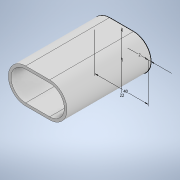
# Autodesk Inventor part: round
Saved by Autodesk Inventor 2022 (Build 260153000, 153)
## iProperties
Created: 2021-10-11
Part Number: round
Material: Generic
Document SubType Name: Modeling
Designer: dangl
Density: 1 g/cm^3
Appearance: Default
Author: dangl
Autodesk Inventor part; units mm, degrees
ref_plane "YZ Plane" through (0, 0, 0) normal (1, 0, 0) x (0, 1, 0)
ref_plane "XZ Plane" through (0, 0, 0) normal (0, 1, 0) x (-1, 0, 0)
ref_plane "XY Plane" through (0, 0, 0) normal (0, 0, 1) x (1, 0, 0)
sketch "Sketch1" plane through (0, 0, 0) normal (0, 0, 1) x (1, 0, 0)
  line L0 (-40, 0) -> (0, 0) construction
  line L1 (-29, 11) -> (-11, 11)
  line L2 (-11, -11) -> (-29, -11)
  arc A0 (-29, 11) -> (-29, -11) centre (-29, 0) ccw
  arc A1 (-11, -11) -> (-11, 11) centre (-11, 0) ccw
  line L3 (-11, 13) -> (-29, 13)
  arc A2 (-29, 13) -> (-29, -13) centre (-29, 0) ccw
  line L4 (-29, -13) -> (-11, -13)
  arc A3 (-11, -13) -> (-11, 13) centre (-11, 0) ccw
  point P0 (-20, 0)
  dimension "d2" = 22
  dimension "d4" = 40
  dimension "d5" = 2
  constraints: 12 end point, 10 point on circle, 4 centre point, 4 tangent, 2 parallel, 2 point on line, 1 horizontal, 1 midpoint, 3 other
  measures "d2" distance between parallel lines of L2 L1
  measures "d4" distance of L0.end L0.start
  measures "d5" radial gap between concentric circles of A1 A3
extrude "Extrusion1" add sketch "Sketch1" along normal blind 3 contours L1 A1 L2 A0 | A3 L4 A2 L3
extrude "Extrusion2" add sketch "Sketch1" along normal blind 63
body "Solid1"
